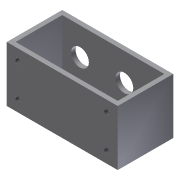
# Autodesk Inventor part: JointC0
Saved by Autodesk Inventor 2011 SP1 (Build 150282100, 282)
## iProperties
Created: 2012-10-16
Part Number: JointC0
Document SubType Name: Modeling
Designer: arihon
Density: 1 g/cm^3
Author: arihon
Autodesk Inventor part; units mm, degrees
ref_plane "YZ Plane" through (0, 0, 0) normal (1, 0, 0) x (0, 1, 0)
ref_plane "XZ Plane" through (0, 0, 0) normal (0, 1, 0) x (-1, 0, 0)
ref_plane "XY Plane" through (0, 0, 0) normal (0, 0, 1) x (1, 0, 0)
sketch "スケッチ1" plane through (0, 0, 0) normal (0, 0, 1) x (1, 0, 0)
  line L0 (-25, 12.5) -> (25, 12.5)
  line L1 (25, 12.5) -> (25, -12.5)
  line L2 (25, -12.5) -> (-25, -12.5)
  line L3 (-25, -12.5) -> (-25, 12.5)
  line L4 (-23, 10.5) -> (23, 10.5)
  line L5 (23, 10.5) -> (23, -10.5)
  line L6 (23, -10.5) -> (-23, -10.5)
  line L7 (-23, -10.5) -> (-23, 10.5)
  point P0 (0, 0)
  dimension "d0" = 50
  dimension "d1" = 25
  dimension "d2" = 12.5
  dimension "d3" = 25
  dimension "d4" = 2
  dimension "d5" = 2
  dimension "d6" = 2
  dimension "d7" = 2
  constraints: 16 end point, 4 parallel, 2 horizontal, 2 perpendicular
  measures "d0" distance of L0.start L0.end
  measures "d1" distance of L2.end L0.start
  measures "d2" distance from line of L0 point (0, 0)
  measures "d3" distance from line of point (0, 0) L3
  measures "d4" distance between parallel lines of L0 L4
  measures "d5" distance between parallel lines of L2 L6
  measures "d6" distance between parallel lines of L1 L5
  measures "d7" distance between parallel lines of L7 L3
extrude "押し出し1" add sketch "スケッチ1" along normal blind 25
sketch "スケッチ4" plane through (-25, -12.5, 0) normal (0, -1, 0) x (1, 0, 0)
  line L0 (50, 25) -> (0, 25) projected
  line L1 (0, 0) -> (0, 25) projected
  line L2 (50, 0) -> (0, 0) projected
  line L3 (50, 0) -> (50, 25) projected
  point P0 (25, 0)
  point P1 (5, 20)
  point P2 (5, 5)
  point P3 (45, 5)
  point P4 (45, 20)
  dimension "d27" = 5
  dimension "d28" = 5
  dimension "d29" = 5
  dimension "d30" = 5
  dimension "d31" = 5
  dimension "d32" = 5
  dimension "d33" = 5
  dimension "d34" = 5
  measures "d27" distance from line of point (5, 20) L0
  measures "d28" distance from line of L1 point (5, 20)
  measures "d29" distance from line of L1 point (5, 5)
  measures "d30" distance from line of L2 point (5, 5)
  measures "d31" distance from line of L0 point (45, 20)
  measures "d32" distance from line of point (45, 20) L3
  measures "d33" distance from line of L2 point (45, 5)
  measures "d34" distance from line of point (45, 5) L3
hole "Hole3" at (-20, -12.5, 20) at (-20, -12.5, 5) at (20, -12.5, 5) at (20, -12.5, 20) direction (0, 1, 0) diameter 2.459 end up to face face through (-7.6667, -10.5, 16.6667) facing (0, 1, 0) thread size "M3x0.5" class "6H" standard "ISO Metric profile"
sketch "スケッチ5" plane through (-25, 12.5, 0) normal (0, 1, 0) x (1, 0, 0)
  line L0 (0, 0) -> (50, 0) projected
  line L1 (0, 0) -> (0, -25) projected
  point P0 (25, 0)
  point P1 (10, -12.5)
  point P2 (30, -12.5)
  dimension "d42" = 10
  dimension "d43" = 20
  dimension "d44" = 12.5
  dimension "d45" = 12.5
  measures "d42" distance from line of L1 point (10, -12.5)
  measures "d43" distance of point (30, -12.5) point (10, -12.5)
  measures "d44" distance from line of point (10, -12.5) L0
  measures "d45" distance from line of point (30, -12.5) L0
hole "Hole4" at (-15, 12.5, 12.5) at (5, 12.5, 12.5) direction (0, -1, 0) diameter 8 end up to face face through (7.6667, 10.5, 8.3333) facing (0, -1, 0)
equation "\"d2\" = 0.5 * d1"
equation "\"d3\" = 0.5 * d0"
equation "\"d5\" = d4"
equation "\"d6\" = d4"
equation "\"d7\" = d4"
equation "\"d28\" = d27"
equation "\"d29\" = d27"
equation "\"d30\" = d27"
equation "\"d31\" = d27"
equation "\"d32\" = d27"
equation "\"d33\" = d27"
equation "\"d34\" = d27"
equation "\"d45\" = d44"
